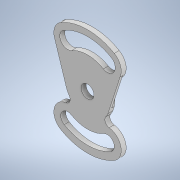
# Autodesk Inventor part: 3.2
Saved by Autodesk Inventor 2020 (Build 240168000, 168)
## iProperties
Created: 2022-03-24
Part Number: 3.2
Material: Типовые
Document SubType Name: Modeling
Designer: guest
Density: 1 g/cm^3
Appearance: По умолчанию
Author: guest
Autodesk Inventor part; units mm, degrees
ref_plane "YZ Plane" through (0, 0, 0) normal (1, 0, 0) x (0, 1, 0)
ref_plane "XZ Plane" through (0, 0, 0) normal (0, 1, 0) x (-1, 0, 0)
ref_plane "XY Plane" through (0, 0, 0) normal (0, 0, 1) x (1, 0, 0)
sketch "Эскиз1" plane through (0, 0, 0) normal (0, 0, 1) x (1, 0, 0)
  circle A0 centre (120.236, 134.1079) radius 13
  arc A1 (165.236, 134.1079) -> (157.0596, 159.9734) centre (120.236, 134.1079) ccw
  arc A2 (168.236, 217.2464) -> (72.236, 217.2464) centre (120.236, 134.1079) ccw
  arc A3 (152.236, 189.5336) -> (88.236, 189.5336) centre (120.236, 134.1079) ccw
  arc A4 (152.236, 189.5336) -> (168.236, 217.2464) centre (160.236, 203.39) ccw
  arc A5 (72.236, 217.2464) -> (88.236, 189.5336) centre (80.236, 203.39) ccw
  arc A6 (174.236, 227.6387) -> (66.236, 227.6387) centre (120.236, 134.1079) ccw
  arc A7 (66.236, 227.6387) -> (52.275, 201.9114) centre (80.236, 203.39) ccw
  line L0 (68.236, 134.1079) -> (172.236, 134.1079)
  arc A8 (75.236, 134.1079) -> (83.4123, 108.2425) centre (120.236, 134.1079) ccw
  arc A9 (52.275, 201.9114) -> (76.5468, 175.6341) centre (80.236, 203.39) ccw
  line L1 (120.236, 242.1079) -> (120.236, 26.1079)
  arc A10 (73.236, 52.7015) -> (167.236, 52.7015) centre (120.236, 134.1079) ccw
  arc A11 (87.236, 76.9503) -> (153.236, 76.9503) centre (120.236, 134.1079) ccw
  arc A12 (87.236, 76.9503) -> (73.236, 52.7015) centre (80.236, 64.8259) ccw
  arc A13 (167.236, 52.7015) -> (153.236, 76.9503) centre (160.236, 64.8259) ccw
  arc A14 (66.236, 40.5772) -> (174.236, 40.5772) centre (120.236, 134.1079) ccw
  arc A15 (174.236, 40.5772) -> (163.9251, 92.5818) centre (160.236, 64.8259) ccw
  arc A16 (76.5468, 92.5818) -> (83.4123, 108.2425) centre (75.2293, 102.4946) ccw
  arc A17 (157.0596, 108.2425) -> (163.9251, 92.5818) centre (165.2426, 102.4946) ccw
  arc A18 (157.0596, 108.2425) -> (165.236, 134.1079) centre (120.236, 134.1079) ccw
  arc A19 (76.5468, 92.5818) -> (66.236, 40.5772) centre (80.236, 64.8259) ccw
  arc A20 (83.4123, 159.9734) -> (76.5468, 175.6341) centre (75.2293, 165.7212) ccw
  arc A21 (83.4123, 159.9734) -> (75.236, 134.1079) centre (120.236, 134.1079) ccw
  arc A22 (163.9251, 175.6341) -> (157.0596, 159.9734) centre (165.2426, 165.7212) ccw
  arc A23 (163.9251, 175.6341) -> (174.236, 227.6387) centre (160.236, 203.39) ccw
  line L2 (161.3771, 115.876) -> (185.8349, 192.0456)
  arc A24 (58.8114, 82.8534) -> (181.6605, 82.8534) centre (120.236, 134.1079) ccw
  arc A25 (181.6605, 185.3625) -> (58.8114, 185.3625) centre (120.236, 134.1079) ccw
  line L3 (120.236, 134.1079) -> (66.236, 40.5772)
  line L4 (120.236, 134.1079) -> (174.236, 40.5772)
  line L5 (120.236, 134.1079) -> (66.236, 227.6387)
  line L6 (120.236, 134.1079) -> (174.236, 227.6387)
  line L7 (53.5661, 194.8626) -> (77.3736, 120.4032)
  point P0 (164.3006, 124.9806)
  point P1 (165.236, 134.1079)
  point P2 (167.2313, 134.1079)
  dimension "d122" = 10
  dimension "d123" = 28
  dimension "d124" = 16
  dimension "d125" = 14
  dimension "d126" = 108
  dimension "d127" = 45
  dimension "d128" = 26
  dimension "d130" = 12.198
  dimension "d131" = 47.802
  dimension "d133" = 0
  dimension "d134" = 4.765
  dimension "d135" = 1.8998
  dimension "d139" = 94.2555
  dimension "d153" = 44.7453
  dimension "d154" = 55.683
  dimension "d155" = 0
  dimension "d156" = 55.683
  dimension "d157" = 0
  dimension "d158" = 81.3984
  dimension "d159" = 1.8998
  dimension "d160" = 77.9423
  dimension "d161" = 0
  dimension "d162" = 85.4495
  dimension "d163" = 89.4905
  dimension "d164" = 0
  dimension "d165" = 89.4905
  constraints: 63 point on circle, 26 centre point, 20 tangent, 16 end point, 9 point on line, 7 coincident, 5 symmetric about line, 2 collinear, 2 equal radius, 1 perpendicular, 1 vertical, 3 other
  measures "d122" radius of A22
  measures "d123" radius of A23
  measures "d124" radius of A4
  measures "d125" radius of A13
  measures "d126" radius of A6
  measures "d127" radius of A21
  measures "d128" diameter of A0
  measures "d130" angle of L6 L2
  measures "d131" angle of L4 L2
  measures "d133" distance from line of A0.centre L0
  measures "d134" distance from line of L0.end L2
  measures "d135" distance from line of A1.start L2
  measures "d139" distance from line of L0.start L2
  measures "d153" distance from line of A0.centre L2
  measures "d154" diameter of L2.end L6
  measures "d155" distance from line of point (185.835, 192.046) L2
  measures "d156" diameter of point (185.835, 192.046) L6
  measures "d157" distance from line of point (167.231, 134.108) L2
  measures "d158" diameter of point (167.231, 134.108) L6
  measures "d159" distance from line of point (165.236, 134.108) L2
  measures "d160" diameter of point (165.236, 134.108) L6
  measures "d161" distance from line of point (164.301, 124.981) L2
  measures "d162" diameter of point (164.301, 124.981) L6
  measures "d163" diameter of L2.start L6
  measures "d164" distance from line of point (161.377, 115.876) L2
  measures "d165" diameter of point (161.377, 115.876) L6
extrude "Выдавливание3" add sketch "Эскиз1" against normal blind 5 contours L0 A18 L2 A17 A15 A24 A13 L4 A0 | A0 L6 A4 A25 A23 A22 A1 L0 | A0 L1 A3 L6 | L4 A11 L1 A0 | A1 A22 A23 L2 L0 | L0 L2 A18 | A0 L5 A3 L1 | L1 A11 L3 A0 | L0 A21 A20 A9 A25 A5 L5 A0 | A0 L3 A12 A24 A19 A16 A8 L0 | A4 L6 A23 A25 | A24 A15 L4 A13 | A8 L7 L0 | L0 L7 A9 A20 A21 | A2 L1 A6 L6 | L4 A14 L1 A10 | A12 L3 A19 A24 | A25 A9 A7 L5 A5 | A2 L5 A6 L1 | L1 A14 L3 A10
extrude "Выдавливание4" add sketch "Эскиз1" against normal blind 10 contours L0 A18 L2 A17 A15 A24 A13 L4 A0 | A0 L6 A4 A25 A23 A22 A1 L0 | A0 L1 A3 L6 | L4 A11 L1 A0 | A0 L5 A3 L1 | L1 A11 L3 A0 | L0 A21 A20 A9 A25 A5 L5 A0 | A0 L3 A12 A24 A19 A16 A8 L0 | A4 L6 A23 A25 | A24 A15 L4 A13 | A2 L1 A6 L6 | L4 A14 L1 A10 | A12 L3 A19 A24 | A25 A9 A7 L5 A5 | A2 L5 A6 L1 | L1 A14 L3 A10
